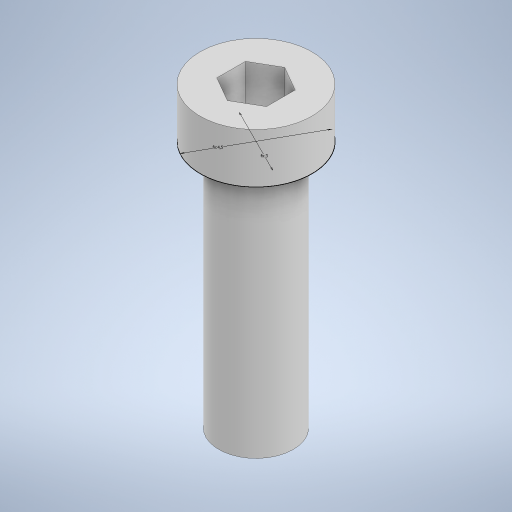
# Autodesk Inventor part: M3 x 10
Saved by Autodesk Inventor 2024.2 (Build 282272000, 272)
## iProperties
Created: 2024-01-31
Part Number: M3 x 10
Material: Generic
Document SubType Name: Modeling
Designer: jp.reyesf
Density: 1 g/cm^3
Appearance: Default
Author: jp.reyesf
Autodesk Inventor part; units mm, degrees
ref_plane "YZ Plane" through (0, 0, 0) normal (1, 0, 0) x (0, 1, 0)
ref_plane "XZ Plane" through (0, 0, 0) normal (0, 1, 0) x (-1, 0, 0)
ref_plane "XY Plane" through (0, 0, 0) normal (0, 0, 1) x (1, 0, 0)
sketch "Sketch1" plane through (0, 0, 0) normal (0, 1, 0) x (-1, 0, 0)
  circle A0 centre (0, 0) radius 2.25
  circle A1 centre (0, 0) radius 1.5
  dimension "d0" = 4.5
  dimension "d1" = 3
  constraints: 2 centre point, 2 coincident
  measures "d0" diameter of A0
  measures "d1" diameter of A1
extrude "Extrusion1" add sketch "Sketch1" against normal blind 10 contours A1
extrude "Extrusion2" add sketch "Sketch1" along normal blind 2 contours A0 | A1
sketch "Sketch2" plane through (0, 2, 0) normal (0, 1, 0) x (1, 0, 0)
  circle A0 centre (0, 0) radius 1.5 projected
  line L0 (-1, -0.5774) -> (-1, 0.5774)
  line L1 (-1, 0.5774) -> (0, 1.1547)
  line L2 (0, 1.1547) -> (1, 0.5774)
  line L3 (1, 0.5774) -> (1, -0.5774)
  line L4 (1, -0.5774) -> (0, -1.1547)
  line L5 (0, -1.1547) -> (-1, -0.5774)
  dimension "d6" = 2
  constraints: 12 end point, 1 coincident, 1 vertical, 13 other
  measures "d6" distance between parallel lines of L3 L0
extrude "Extrusion3" cut sketch "Sketch2" against normal blind 1.5 contours L0 L1 L2 L3 L4 L5
equation "\"d0\" = D_"
equation "\"d1\" = M_"
equation "\"d2\" = L_"
equation "\"d4\" = K_"
equation "\"d6\" = S_"
equation "\"d7\" = t_"
equation "\"K_\" = 2"
equation "\"D_\" = 4.5"
equation "\"S_\" = 2"
equation "\"t_\" = 1.5"
equation "\"M_\" = 3"
equation "\"L_\" = 10"
body "Solid1"
